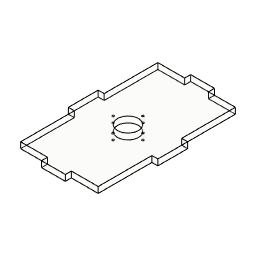
ASM_asian_hornet_trap (Autodesk Fusion 360 archive; units mm, degrees)
design "bottom_plate"
Autodesk Fusion 360 part; units mm, degrees
sketch "Esquisse1" plane through (0, 0, 0) normal (0, 0, 1) x (1, 0, 0)
  line L0 (75, -125) -> (-75, -125) construction
  line L1 (-75, -125) -> (-75, 125) construction
  line L2 (-75, 125) -> (75, 125) construction
  line L3 (75, 125) -> (75, -125) construction
  line L4 (75, -125) -> (-75, 125) construction
  line L5 (-75, -125) -> (75, 125) construction
  circle A0 centre (0, 0) radius 17.5
  circle A1 centre (0, 0) radius 25 construction
  circle A2 centre (0, 25) radius 1.6
  circle A3 centre (-25, 0) radius 1.6
  circle A4 centre (0, -25) radius 1.6
  circle A5 centre (25, 0) radius 1.6
  line L6 (0, 125) -> (0, -125)
  line L7 (-75, 0) -> (75, 0)
  line L8 (75, 125) -> (-75, 125) construction
  line L9 (-75, -125) -> (75, -125) construction
  line L10 (75, -125) -> (-75, -125) construction
  line L11 (-65, 115) -> (-65, 25)
  line L12 (-65, 25) -> (-75, 25)
  line L13 (-75, 25) -> (-75, -25)
  line L14 (-75, -25) -> (-65, -25)
  line L15 (-65, -25) -> (-65, -115)
  line L16 (65, 115) -> (65, 25)
  line L17 (65, 25) -> (75, 25)
  line L18 (75, -125) -> (75, 125) construction
  line L19 (75, -25) -> (65, -25)
  line L20 (65, -25) -> (65, -115)
  line L21 (75, 25) -> (75, -25)
  line L22 (-65, 115) -> (-20, 115)
  line L23 (-20, 115) -> (-20, 125)
  line L24 (20, 125) -> (-20, 125)
  line L25 (20, 125) -> (20, 115)
  line L26 (20, 115) -> (65, 115)
  line L27 (20, -125) -> (20, -115)
  line L28 (20, -115) -> (65, -115)
  line L29 (20, -125) -> (-20, -125)
  line L30 (-20, -115) -> (-20, -125)
  line L31 (-65, -115) -> (-20, -115)
  circle A6 centre (0, 0) radius 33.25 construction
  dimension "d1" = 150
  dimension "d2" = 250
  dimension "d3" = 35
  dimension "d5" = 3.2
  dimension "d9" = 50
  dimension "d14" = 40
  dimension "d15" = 10
  dimension "d16" = 10
  dimension "d17" = 66.5
  dimension "d18" = 50
  constraint horizontal L0
  constraint perpendicular L0 L1
  constraint parallel L0 L2
  constraint parallel L1 L3
  constraint coincident L4 A0.centre
  constraint coincident L5 A0.centre
  constraint coincident A0.centre A1.centre
  constraint coincident A1 A2.centre
  constraint coincident A1 A4.centre
  constraint coincident A1 A5.centre
  constraint equal A2 A5
  constraint equal A4 A5
  constraint equal A3 A4
  constraint midpoint L2 L6.start
  constraint midpoint L0 L6.end
  constraint midpoint L1 L7.start
  constraint midpoint L3 L7.end
  constraint coincident A2.centre L6
  constraint coincident A5.centre L7
  constraint coincident A4.centre L6
  constraint coincident A3.centre L7
  constraint coincident A1 A3.centre
  constraint symmetric L1.end L6 L2.end
  constraint symmetric L2.end L6 L1.end
  constraint symmetric L1.end L7 L0.end
  constraint symmetric L2.end L7 L0.start
  constraint symmetric L7 L2.end L0.start
  constraint symmetric L7 L1.end L0.end
  constraint perpendicular L8 L11
  constraint coincident L1 L12.end
  constraint perpendicular L1 L12
  constraint coincident L1 L13.end
  constraint perpendicular L13 L14
  constraint equal L12 L14
  constraint vertical L15
  constraint symmetric L7 L11.end L14.end
  constraint symmetric L0.end L6 L0.start
  constraint symmetric L6 L11.end L16.end
  constraint symmetric L6 L12.end L17.end
  constraint symmetric L6 L13.end L19.start
  constraint symmetric L6 L14.end L19.end
  constraint perpendicular L11 L22
  constraint coincident L8 L23.end
  constraint perpendicular L8 L23
  constraint coincident L2 L24.start
  constraint perpendicular L23 L24
  constraint perpendicular L24 L25
  constraint perpendicular L16 L26
  constraint symmetric L6 L23.end L24.start
  constraint equal L23 L25
  constraint vertical L16
  constraint symmetric L7 L11.start L15.end
  constraint symmetric L7 L22.end L30.start
  constraint symmetric L7 L23.end L29.end
  constraint symmetric L7 L24.start L27.start
  constraint symmetric L7 L25.end L27.end
  constraint symmetric L7 L16.start L20.end
  measures "d1" distance of L1.end L2.end
  measures "d2" distance of L0.end L1.end
  measures "d3" diameter of A0
  measures "d5" diameter of A2
  measures "d9" distance of L12 L14
  measures "d14" distance of L23 L25
  measures "d15" distance of L8 L22
  measures "d16" distance of L1 L11
  measures "d17" diameter of A6
  measures "d18" diameter of A1
extrude "Extrusion1" add sketch "Esquisse1" along normal blind 10 contours A0 A4 A5 L6 L7 L19 L20 L21 L27 L28 L29 | A0 A2 A5 L6 L7 L16 L17 L21 L24 L25 L26 | A0 A2 A3 L6 L7 L11 L12 L13 L22 L23 L24 | A0 A3 A4 L6 L7 L13 L14 L15 L29 L30 L31

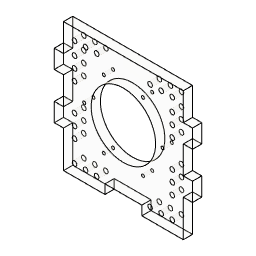
design "front_and_back_plate"
Autodesk Fusion 360 part; units mm, degrees
sketch "Esquisse1" plane through (0, 0, 0) normal (0, 1, 0) x (1, 0, 0)
  line L0 (75, 75) -> (-75, 75) construction
  line L1 (-75, 75) -> (-75, -75) construction
  line L2 (-75, -75) -> (75, -75) construction
  line L3 (75, -75) -> (75, 75) construction
  line L4 (75, 75) -> (-75, -75) construction
  line L5 (-75, 75) -> (75, -75) construction
  circle A0 centre (0, 0) radius 35
  circle A1 centre (0, 0) radius 42.5 construction
  circle A2 centre (42.5, 0) radius 1.6
  line L6 (42.5, 0) -> (21.25, 36.8061) construction
  line L7 (21.25, 36.8061) -> (-21.25, 36.8061) construction
  line L8 (-21.25, 36.8061) -> (-42.5, 0) construction
  line L9 (-42.5, 0) -> (-21.25, -36.8061) construction
  line L10 (-21.25, -36.8061) -> (21.25, -36.8061) construction
  line L11 (21.25, -36.8061) -> (42.5, 0) construction
  circle A3 centre (21.25, -36.8061) radius 1.6
  circle A4 centre (-21.25, -36.8061) radius 1.6
  circle A5 centre (-42.5, 0) radius 1.6
  circle A6 centre (-21.25, 36.8061) radius 1.6
  circle A7 centre (21.25, 36.8061) radius 1.6
  line L12 (-65, -65) -> (0, -65)
  line L13 (0, -75) -> (0, 75)
  line L14 (-75, 0) -> (75, 0)
  line L15 (65, -65) -> (0, -65)
  line L16 (-65, 65) -> (0, 65) construction
  line L17 (65, 65) -> (0, 65) construction
  line L18 (-65, 35) -> (-65, 65)
  line L19 (-65, 35) -> (-75, 35)
  line L20 (-75, -75) -> (-75, 75) construction
  line L21 (-75, 15) -> (-65, 15)
  line L22 (-65, 15) -> (-65, 0.2731)
  line L23 (75, 75) -> (75, -75) construction
  line L24 (-75, 15) -> (-75, 35)
  line L25 (-65, -65) -> (-65, -35)
  line L26 (-65, -35) -> (-75, -35)
  line L27 (-75, -15) -> (-65, -15)
  line L28 (-65, -15) -> (-65, 0.2731)
  line L29 (-65, -65) -> (-65, 75) construction
  line L30 (-75, -15) -> (-75, -35)
  line L31 (65, -15) -> (65, 0.2731)
  line L32 (65, -65) -> (65, -35)
  line L33 (75, 15) -> (75, 35)
  line L34 (65, 35) -> (75, 35)
  line L35 (75, -15) -> (75, -35)
  line L36 (75, 15) -> (65, 15)
  line L37 (65, 15) -> (65, 0.2731)
  line L38 (65, -35) -> (75, -35)
  line L39 (65, 35) -> (65, 65)
  line L40 (75, -15) -> (65, -15)
  line L41 (-65, 65) -> (-65, 75)
  line L42 (-65, 75) -> (-20, 75)
  line L43 (-20, 75) -> (-20, 65)
  line L44 (-20, 65) -> (20, 65)
  line L45 (20, 65) -> (20, 75)
  line L46 (20, 75) -> (65, 75)
  line L47 (65, 75) -> (65, 65)
  circle A8 centre (0, 0) radius 50 construction
  point P0 (75, 0)
  point P1 (-75, -25)
  point P2 (-75, 25)
  dimension "d1" = 150
  dimension "d2" = 150
  dimension "d3" = 70
  dimension "d4" = 7.5
  dimension "d5" = 3.2
  dimension "d9" = 10
  dimension "d22" = 20
  dimension "d24" = 20
  dimension "d25" = 10
  dimension "d32" = 40
  dimension "d56" = 15
  dimension "d58" = 50
  constraint horizontal L0
  constraint perpendicular L0 L1
  constraint parallel L1 L3
  constraint coincident L4 A0.centre
  constraint coincident L5 A0.centre
  constraint coincident A0.centre A1.centre
  constraint concentric A0 A1
  constraint coincident A1 A2.centre
  constraint coincident A2.centre L6.start
  constraint coincident L10.end L11.start
  constraint coincident L9.end L10.start
  constraint coincident L8.end L9.start
  constraint coincident L7.end L8.start
  constraint coincident L6.end L7.start
  constraint equal A3 A4
  constraint equal A4 A5
  constraint equal A5 A6
  constraint equal A6 A7
  constraint equal A2 A7
  constraint perpendicular L1 L12
  constraint midpoint L2 L13.start
  constraint midpoint L0 L13.end
  constraint midpoint L1 L14.start
  constraint midpoint L3 P0
  constraint symmetric L12.start L13 L15.start
  constraint symmetric L12.end L13 L15.end
  constraint symmetric L0.start L14 L2.end
  constraint symmetric L0.end L14 L1.end
  constraint symmetric L1.end L14 L0.end
  constraint symmetric L2.end L14 L0.start
  constraint symmetric L12.start L14 L16.start
  constraint symmetric L12.end L14 L16.end
  constraint symmetric L14 L15.start L17.start
  constraint symmetric L14 L12.end L16.end
  constraint coincident A2.centre L14
  constraint perpendicular L12 L25
  constraint coincident L1 L26.end
  constraint perpendicular L1 L26
  constraint coincident L1 L27.start
  constraint perpendicular L1 L27
  constraint perpendicular L14 L28
  constraint coincident L0 L29.end
  constraint perpendicular L0 L29
  constraint coincident L12.start L28
  constraint vertical L24
  constraint coincident L1 L21.start
  constraint symmetric L13 L14.start P0
  constraint symmetric L13 L16.start L17.start
  constraint symmetric L13 L18.start L34.start
  constraint symmetric L13 L19.end L33.end
  constraint symmetric L13 L21.start L33.start
  constraint symmetric L13 L21.end L36.end
  constraint symmetric L13 L22.end L31.end
  constraint symmetric L13 L25.end L32.end
  constraint symmetric L13 L26.end L35.end
  constraint symmetric L13 L27.start L35.start
  constraint symmetric L13 L27.end L31.start
  constraint vertical L22
  constraint coincident L0 L42.end
  constraint coincident L16 L43.end
  constraint perpendicular L16 L43
  constraint coincident L17 L44.end
  constraint perpendicular L43 L44
  constraint coincident L0 L45.end
  constraint perpendicular L0 L45
  constraint coincident L0 L46.end
  constraint perpendicular L17 L47
  constraint symmetric L13 L43.end L44.end
  constraint vertical L18
  constraint concentric A1 A8
  constraint symmetric L14 L21.end L27.end
  constraint midpoint L30 P1
  constraint midpoint L24 P2
  measures "d1" distance of L1.end L2.end
  measures "d2" distance of L0.end L1.end
  measures "d3" diameter of A0
  measures "d4" distance of A0 A1
  measures "d5" diameter of A3
  measures "d9" distance of L2 L12
  measures "d22" distance of L19 L21
  measures "d24" distance of L26 L27
  measures "d25" distance of L20 L29
  measures "d32" distance of L43 L45
  measures "d56" distance of A0 A8
  measures "d58" distance of P1 P2
extrude "Extrusion1" add sketch "Esquisse1" along normal blind 10 contours A0 A2 L13 L14 L15 L31 L32 L35 L38 L40 | A0 A2 L13 L14 L31 L33 L34 L36 L37 L39 L44 L45 L46 L47 | A0 A5 L13 L14 L18 L19 L21 L22 L24 L28 L41 L42 L43 L44 | A0 A5 L12 L13 L14 L25 L26 L27 L28 L30
sketch "Esquisse3" plane through (0, 0, 0) normal (0, -1, 0) x (1, 0, 0)
  line L0 (65, 65) -> (-65, 65)
  line L1 (-65, 65) -> (-65, 35)
  line L2 (-65, 35) -> (-75, 35)
  line L3 (-75, 35) -> (-75, 15)
  line L4 (-75, 15) -> (-65, 15)
  line L5 (-65, 15) -> (-65, -15)
  line L6 (-65, -15) -> (-75, -15)
  line L7 (-75, -15) -> (-75, -35)
  line L8 (-75, -35) -> (-65, -35)
  line L9 (-65, -35) -> (-65, -75)
  line L10 (-65, -75) -> (-20, -75)
  line L11 (-20, -75) -> (-20, -65)
  line L12 (-20, -65) -> (20, -65)
  line L13 (20, -65) -> (20, -75)
  line L14 (20, -75) -> (65, -75)
  line L15 (65, -75) -> (65, -35)
  line L16 (65, -35) -> (75, -35)
  line L17 (75, -35) -> (75, -15)
  line L18 (75, -15) -> (65, -15)
  line L19 (65, -15) -> (65, 15)
  line L20 (65, 15) -> (75, 15)
  line L21 (75, 15) -> (75, 35)
  line L22 (75, 35) -> (65, 35)
  line L23 (65, 35) -> (65, 65)
  circle A0 centre (-42.5, 0) radius 1.6
  circle A1 centre (21.25, 36.8061) radius 1.6
  circle A2 centre (21.25, -36.8061) radius 1.6
  circle A3 centre (-21.25, -36.8061) radius 1.6
  circle A4 centre (42.5, 0) radius 1.6
  circle A5 centre (-21.25, 36.8061) radius 1.6
  circle A6 centre (0, 0) radius 35
  line L24 (-65, -64.8) -> (65, -64.8) construction
  line L25 (-65, -62.3) -> (65, -62.3) construction
  circle A7 centre (-53, -62.3) radius 2.5
  circle A8 centre (-41, -62.3) radius 2.5
  circle A9 centre (-29, -62.3) radius 2.5
  line L26 (0, -64.8) -> (0, 65)
  circle A10 centre (41, -62.3) radius 2.5
  circle A11 centre (53, -62.3) radius 2.5
  circle A12 centre (29, -62.3) radius 2.5
  line L27 (-53, -75) -> (-53, 65) construction
  circle A13 centre (-53, -39) radius 2.5
  circle A14 centre (-53, -27) radius 2.5
  circle A15 centre (-53, -15) radius 2.5
  circle A16 centre (-53, 15) radius 2.5
  circle A17 centre (-53, 27) radius 2.5
  circle A18 centre (-53, 39) radius 2.5
  line L28 (-65, 0) -> (65, 0)
  circle A19 centre (53, -15) radius 2.5
  circle A20 centre (53, 39) radius 2.5
  circle A21 centre (53, -39) radius 2.5
  circle A22 centre (53, 15) radius 2.5
  circle A23 centre (53, 27) radius 2.5
  circle A24 centre (53, -27) radius 2.5
  line L29 (53, -75) -> (53, 65) construction
  line L30 (-53, 53) -> (53, 53) construction
  circle A25 centre (-53, 53) radius 2.5
  circle A26 centre (-41, 53) radius 2.5
  circle A27 centre (-29, 53) radius 2.5
  line L31 (-41, 53) -> (-41, -62.3) construction
  line L32 (-29, 53) -> (-29, -62.3) construction
  circle A28 centre (53, 53) radius 2.5
  circle A29 centre (29, 53) radius 2.5
  circle A30 centre (41, 53) radius 2.5
  circle A31 centre (0, 0) radius 50 construction
  point P0 (41, 53)
  point P1 (53, 53)
  point P2 (29, 53)
  dimension "d33" = 0.2
  dimension "d34" = 5
  dimension "d36" = 12
  dimension "d37" = 12
  dimension "d38" = 12
  dimension "d39" = 5
  dimension "d40" = 5
  dimension "d41" = 5
  dimension "d42" = 5
  dimension "d43" = 5
  dimension "d44" = 5
  dimension "d45" = 12
  dimension "d46" = 12
  dimension "d47" = 12
  dimension "d48" = 12
  dimension "d49" = 30
  dimension "d50" = 12
  dimension "d51" = 5
  dimension "d52" = 5
  dimension "d53" = 5
  dimension "d54" = 12
  dimension "d57" = 15
  constraint coincident L9 L24.start
  constraint coincident L15 L24.end
  constraint perpendicular L15 L24
  constraint coincident L9 L25.start
  constraint coincident L15 L25.end
  constraint perpendicular L15 L25
  constraint coincident L25 A7.centre
  constraint coincident L25 A8.centre
  constraint coincident L25 A9.centre
  constraint equal A8 A9
  constraint equal A7 A8
  constraint tangent L24 A7
  constraint midpoint L24 L26.start
  constraint midpoint L0 L26.end
  constraint symmetric A7 L26 A11
  constraint symmetric A8 L26 A10
  constraint symmetric A9 L26 A12
  constraint coincident L10 L27.start
  constraint coincident L0 L27.end
  constraint perpendicular L0 L27
  constraint coincident L27 A13.centre
  constraint coincident L27 A14.centre
  constraint coincident L27 A15.centre
  constraint coincident L27 A16.centre
  constraint coincident L27 A17.centre
  constraint coincident L27 A18.centre
  constraint midpoint L5 L28.start
  constraint midpoint L19 L28.end
  constraint symmetric A15.centre A16.centre L28
  constraint symmetric L26 L27.start L29.start
  constraint symmetric L26 L27.end L29.end
  constraint symmetric L26 A13 A21
  constraint symmetric L26 A14 A24
  constraint symmetric L26 A15 A19
  constraint symmetric L26 A16 A22
  constraint symmetric L26 A17 A23
  constraint symmetric L26 A18 A20
  constraint coincident L27 L30.start
  constraint coincident L29 P1
  constraint perpendicular L29 L30
  constraint coincident L30.start A25.centre
  constraint coincident L30 A26.centre
  constraint coincident L30 A27.centre
  constraint coincident A26.centre L31.start
  constraint coincident A8.centre L31.end
  constraint coincident A27.centre L32.start
  constraint coincident A9.centre L32.end
  constraint vertical L32
  constraint vertical L31
  constraint symmetric L26 L30.start P1
  constraint symmetric L26 A25 A28
  constraint symmetric L26 A26 A30
  constraint symmetric L26 A27 A29
  constraint symmetric L26 A26.centre P0
  constraint symmetric L26 A27.centre P2
  constraint coincident A6.centre A31.centre
  measures "d33" distance of L12 L24
  measures "d34" diameter of A7
  measures "d36" distance of A7.centre A8.centre
  measures "d37" distance of A8.centre A9.centre
  measures "d38" distance of L25.start A7.centre
  measures "d39" diameter of A13
  measures "d40" diameter of A14
  measures "d41" diameter of A15
  measures "d42" diameter of A16
  measures "d43" diameter of A17
  measures "d44" diameter of A18
  measures "d45" distance of A13.centre A14.centre
  measures "d46" distance of A14.centre A15.centre
  measures "d47" distance of A16.centre A17.centre
  measures "d48" distance of A17.centre A18.centre
  measures "d49" distance of A15.centre A16.centre
  measures "d50" distance of L1 L27
  measures "d51" diameter of A25
  measures "d52" diameter of A26
  measures "d53" diameter of A27
  measures "d54" distance of L0 L30
  measures "d57" distance of A6 A31
extrude "Extrusion3" cut sketch "Esquisse3" against normal through all contours A7 | A8 | A9 | A10 | A11 | A12 | A13 | A14 | A15 | A16 | A17 | A18 | A19 | A20 | A21 | A22 | A23 | A24 | A25 | A26 | A27 | A28 | A29 | A30

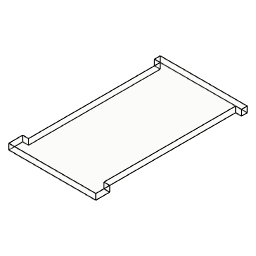
design "top_plate"
Autodesk Fusion 360 part; units mm, degrees
sketch "Esquisse1" plane through (0, 0, 0) normal (0, 0, 1) x (1, 0, 0)
  line L0 (75, -125) -> (-75, -125) construction
  line L1 (-75, -125) -> (-75, 125) construction
  line L2 (-75, 125) -> (75, 125) construction
  line L3 (75, 125) -> (75, -125) construction
  line L4 (75, -125) -> (-75, 125) construction
  line L5 (-75, -125) -> (75, 125) construction
  line L6 (-75, 125) -> (75, 125) construction
  line L7 (75, 125) -> (75, 136) construction
  line L8 (75, 136) -> (-75, 136) construction
  line L9 (-75, 136) -> (-75, 125) construction
  line L10 (-75, 136) -> (-75, 126)
  line L11 (-75, 126) -> (-65, 126)
  line L12 (-65, 126) -> (-65, -101)
  line L13 (-65, -101) -> (-75, -101)
  line L14 (-75, -101) -> (-75, -125)
  line L15 (-75, -125) -> (0, -125)
  line L16 (0, -125) -> (0, -120)
  line L17 (0, -120) -> (0, 136)
  line L18 (-75, 136) -> (0, 136)
  line L19 (75, 136) -> (0, 136)
  line L20 (75, 136) -> (75, 125) construction
  line L21 (0, -120) -> (0, 136)
  line L22 (0, -125) -> (0, -120)
  line L23 (75, -101) -> (75, -125)
  line L24 (75, -125) -> (0, -125)
  line L25 (65, -101) -> (75, -101)
  line L26 (75, -125) -> (75, 125) construction
  line L27 (75, 126) -> (65, 126)
  line L28 (75, 136) -> (75, 126)
  line L29 (65, 126) -> (65, -101)
  dimension "d1" = 150
  dimension "d2" = 250
  dimension "d3" = 11
  dimension "d4" = 10
  dimension "d5" = 10
  dimension "d6" = 24
  constraint horizontal L0
  constraint perpendicular L0 L1
  constraint parallel L0 L2
  constraint parallel L1 L3
  constraint coincident L4 origin
  constraint coincident L5 origin
  constraint horizontal L6
  constraint vertical L7
  constraint horizontal L8
  constraint vertical L9
  constraint coincident L9 L10.end
  constraint perpendicular L2 L10
  constraint perpendicular L10 L11
  constraint perpendicular L2 L12
  constraint coincident L1 L13.end
  constraint perpendicular L1 L13
  constraint midpoint L0 L15.end
  constraint perpendicular L0 L16
  constraint midpoint L8 L17.end
  constraint perpendicular L8 L17
  constraint symmetric L0.end L17 L0.start
  constraint symmetric L1.end L17 L2.end
  constraint symmetric L8.end L17 L7.end
  constraint symmetric L10.end L17 L27.start
  constraint symmetric L11.end L17 L27.end
  constraint symmetric L12.end L17 L25.start
  constraint symmetric L13.end L17 L23.start
  constraint symmetric L15.end L17 L16.start
  constraint symmetric L16.end L17 L21.start
  constraint symmetric L18.end L17 L19.end
  measures "d1" distance of L0.start L0.end
  measures "d2" distance of L0.start L2.end
  measures "d3" distance of L1.end L8.end
  measures "d4" distance of L10.end L11.end
  measures "d5" distance of L8 L11
  measures "d6" distance of L13 L15
extrude "Extrusion1" add sketch "Esquisse1" along normal blind 10

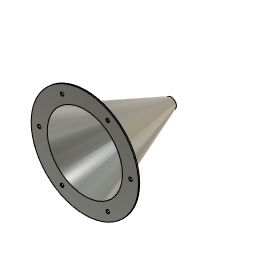
design "cone"
Autodesk Fusion 360 part; units mm, degrees
sketch "Esquisse1" plane through (0, 0, 0) normal (0, 0, 1) x (1, 0, 0)
  line L0 (0, 0) -> (0, 80)
  line L1 (0, 0) -> (50, 0) construction
  line L2 (50, 0) -> (50, 1)
  line L3 (50, 1) -> (35.685, 1)
  line L4 (35.685, 1) -> (4.9324, 80.3613)
  line L5 (4, 80) -> (35, 0)
  line L6 (35, 0) -> (50, 0)
  line L7 (4.9324, 80.3613) -> (4, 80)
  line L8 (4, 80) -> (0, 80) construction
  dimension "d1" = 1
  dimension "d2" = 35
  dimension "d3" = 15
  dimension "d4" = 4
  dimension "d5" = 80
  constraint coincident L0.start L1.start
  constraint vertical L0
  constraint perpendicular L0 L1
  constraint perpendicular L1 L2
  constraint perpendicular L2 L3
  constraint coincident L1 L5.end
  constraint parallel L4 L5
  constraint perpendicular L5 L7
  constraint horizontal L8
  constraint equal L2 L7
  measures "d1" distance of L1.end L2.end
  measures "d2" distance of L0.start L5.end
  measures "d3" distance of L1.end L5.end
  measures "d4" distance of L0.end L5.start
  measures "d5" distance of L0.start L0.end
revolve "Révolution1" add sketch "Esquisse1" angle 360 about axis through (0, 0, 0) along (0, 1, 0)
sketch "Esquisse2" plane through (0, 0, 0) normal (0, -1, 0) x (1, 0, 0)
  circle A0 centre (0, 0) radius 50
  circle A1 centre (0, 0) radius 35
  line L0 (21.25, 36.8061) -> (-21.25, 36.8061) construction
  line L1 (-21.25, 36.8061) -> (-42.5, 0) construction
  line L2 (-42.5, 0) -> (-21.25, -36.8061) construction
  line L3 (-21.25, -36.8061) -> (21.25, -36.8061) construction
  line L4 (21.25, -36.8061) -> (42.5, 0) construction
  line L5 (42.5, 0) -> (21.25, 36.8061) construction
  line L6 (-50, 0) -> (50, 0) construction
  circle A2 centre (0, 0) radius 42.5 construction
  circle A3 centre (-21.25, 36.8061) radius 1.6
  circle A4 centre (21.25, 36.8061) radius 1.6
  circle A5 centre (42.5, 0) radius 1.6
  circle A6 centre (21.25, -36.8061) radius 1.6
  circle A7 centre (-21.25, -36.8061) radius 1.6
  circle A8 centre (-42.5, 0) radius 1.6
  dimension "d7" = 7.5
  dimension "d8" = 3.2
  constraint coincident A0.centre A1.centre
  constraint coincident A0 L6.start
  constraint coincident A0 L6.end
  constraint horizontal L6
  constraint coincident L4.end L6
  constraint coincident A0.centre L6
  constraint coincident L0.end A2
  constraint coincident L0.end L1.start
  constraint coincident L0.start L5.end
  constraint coincident L4.end L5.start
  constraint coincident L3.end L4.start
  constraint coincident L2.end L3.start
  constraint coincident L1.end L2.start
  constraint equal A3 A4
  constraint equal A4 A5
  constraint equal A5 A6
  constraint equal A6 A7
  constraint equal A7 A8
  measures "d7" distance of A1 A2
  measures "d8" diameter of A3
extrude "Extrusion1" cut sketch "Esquisse2" against normal through all contours A3 | A4 | A5 | A6 | A7 | A8
equation "d2 = ( 70 / 2 ) * 1 mm"

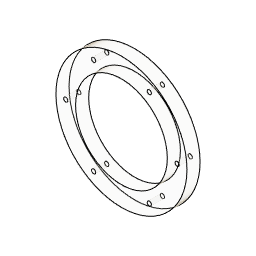
design "cone_fastener"
Autodesk Fusion 360 part; units mm, degrees
sketch "Esquisse1" plane through (0, 0, 0) normal (0, 1, 0) x (1, 0, 0)
  circle A0 centre (0, 0) radius 35
  circle A1 centre (0, 0) radius 50
  line L0 (42.5, 0) -> (21.25, 36.8061) construction
  line L1 (21.25, 36.8061) -> (-21.25, 36.8061) construction
  line L2 (-21.25, 36.8061) -> (-42.5, 0) construction
  line L3 (-42.5, 0) -> (-21.25, -36.8061) construction
  line L4 (-21.25, -36.8061) -> (21.25, -36.8061) construction
  line L5 (21.25, -36.8061) -> (42.5, 0) construction
  circle A2 centre (0, 0) radius 42.5 construction
  line L6 (50, 0) -> (-50, 0)
  line L7 (0, -50) -> (0, 50)
  circle A3 centre (21.25, -36.8061) radius 1.6
  circle A4 centre (-21.25, -36.8061) radius 1.6
  circle A5 centre (-42.5, 0) radius 1.6
  circle A6 centre (-21.25, 36.8061) radius 1.6
  circle A7 centre (21.25, 36.8061) radius 1.6
  circle A8 centre (42.5, 0) radius 1.6
  dimension "d1" = 70
  dimension "d2" = 15
  dimension "d5" = 7.5
  dimension "d6" = 3.2
  constraint coincident A0.centre A1.centre
  constraint coincident L4.end A2
  constraint coincident A1 L6.start
  constraint coincident A1 L6.end
  constraint horizontal L6
  constraint coincident A1 L7.start
  constraint coincident A1 L7.end
  constraint perpendicular L6 L7
  constraint coincident L0.start L6
  constraint coincident L4.end L5.start
  constraint coincident L3.end L4.start
  constraint coincident A0.centre L6
  constraint coincident L2.end L3.start
  constraint coincident L1.end L2.start
  constraint coincident L0.end L1.start
  constraint coincident L0.start L5.end
  constraint equal A3 A4
  constraint equal A3 A8
  constraint equal A7 A8
  constraint equal A4 A5
  constraint equal A6 A7
  measures "d1" diameter of A0
  measures "d2" distance of A0 A1
  measures "d5" distance of A0 A2
  measures "d6" diameter of A4
extrude "Extrusion1" add sketch "Esquisse1" along normal blind 10 contours A0 A1 L6 L7 A8 | A0 A1 L6 L7 A8 | A0 A1 L6 L7 A5 | A0 A1 L6 L7 A5

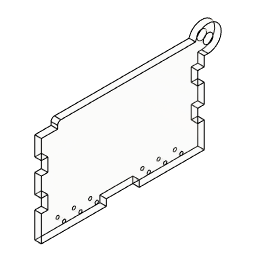
design "right_and_left_plate"
Autodesk Fusion 360 part; units mm, degrees
sketch "Esquisse1" plane through (0, 0, 0) normal (1, 0, 0) x (0, 1, 0)
  line L0 (0, 0) -> (-250, 0) construction
  line L1 (-250, 0) -> (-250, 150) construction
  line L2 (-220, 150) -> (0, 150) construction
  line L3 (0, 150) -> (0, 0) construction
  line L4 (0, 0) -> (0, 39.75)
  line L5 (-10, 39.75) -> (0, 39.75)
  line L6 (-10, 39.75) -> (-10, 60.25)
  line L7 (-10, 60.25) -> (0, 60.25)
  line L8 (0, 60.25) -> (0, 89.75)
  line L9 (-10, 89.75) -> (-10, 110.25)
  line L10 (-10, 110.25) -> (0, 110.25)
  line L11 (-10, 89.75) -> (0, 89.75)
  line L12 (0, 110.25) -> (0, 125)
  line L13 (-13.3649, 150) -> (-250, 150) construction
  line L14 (11, 150) -> (1, 150) construction
  line L15 (1, 150) -> (1, 140) construction
  line L16 (1, 140) -> (11, 140) construction
  line L17 (11, 140) -> (11, 150) construction
  line L18 (11, 150) -> (1, 140) construction
  line L19 (1, 150) -> (11, 140) construction
  arc A0 (6, 125) -> (-13.3649, 150) centre (6, 145) ccw
  line L20 (-13.3649, 150) -> (-220, 150)
  line L21 (-250, 140) -> (-250, 110.5)
  line L22 (-250, 110.5) -> (-240, 110.5)
  line L23 (-240, 110.5) -> (-240, 90)
  line L24 (-240, 90) -> (-250, 90)
  line L25 (-250, 90) -> (-250, 60.5)
  line L26 (-250, 60.5) -> (-240, 60.5)
  line L27 (-240, 60.5) -> (-240, 40)
  line L28 (-240, 40) -> (-250, 40)
  line L29 (-250, 40) -> (-250, 0)
  line L30 (-250, 0) -> (-150.25, 0)
  line L31 (-150.25, 0) -> (-150.25, 10)
  line L32 (-150.25, 10) -> (-99.75, 10)
  line L33 (-99.75, 10) -> (-99.75, 0)
  line L34 (-99.75, 0) -> (0, 0)
  line L35 (-125, 150) -> (-125, 10) construction
  line L36 (-250, 75) -> (0, 75) construction
  circle A1 centre (6, 145) radius 7.5
  circle A2 centre (6, 145) radius 7.0711 construction
  line L37 (-125, 150) -> (-125, 0) construction
  line L38 (-225, 145) -> (-225, 140)
  line L39 (-225, 140) -> (-250, 140)
  line L40 (0, 140) -> (-250, 140) construction
  line L41 (0, 125) -> (6, 125)
  arc A3 (6, 125) -> (0, 125.9212) centre (6, 145) ccw construction
  arc A4 (0, 125.9212) -> (6, 125) centre (6, 145) ccw construction
  arc A5 (-220, 150) -> (-225, 145) centre (-220, 145) ccw
  point P0 (6, 145)
  point P1 (-10, 100)
  point P2 (-10, 50)
  dimension "d1" = 250
  dimension "d2" = 150
  dimension "d4" = 20.5
  dimension "d7" = 10
  dimension "d8" = 40
  dimension "d11" = 10
  dimension "d12" = 10
  dimension "d13" = 40
  dimension "d29" = 50.5
  dimension "d30" = 10
  dimension "d36" = 140
  dimension "d37" = 10
  dimension "d38" = 1
  dimension "d40" = 5
  dimension "d41" = 50
  dimension "d42" = 15
  dimension "d43" = 25
  constraint horizontal L0
  constraint vertical L1
  constraint horizontal L2
  constraint vertical L3
  constraint coincident L0.start L3.end
  constraint coincident L3 L4.end
  constraint perpendicular L3 L5
  constraint perpendicular L5 L6
  constraint coincident L3 L7.end
  constraint perpendicular L3 L7
  constraint coincident L3 L8.end
  constraint perpendicular L7 L9
  constraint coincident L3 L10.end
  constraint perpendicular L3 L10
  constraint perpendicular L3 L11
  constraint coincident L3 A3.end
  constraint equal L7 L11
  constraint coincident L13.start A3
  constraint coincident L2 L13.start
  constraint horizontal L14
  constraint perpendicular L14 L15
  constraint parallel L14 L16
  constraint parallel L15 L17
  constraint coincident L18 P0
  constraint coincident L19 P0
  constraint coincident P0 A0.centre
  constraint equal A0 A3
  constraint coincident L1 L21.end
  constraint perpendicular L21 L22
  constraint perpendicular L22 L23
  constraint coincident L1 L24.end
  constraint perpendicular L1 L24
  constraint coincident L1 L25.end
  constraint perpendicular L1 L26
  constraint perpendicular L26 L27
  constraint coincident L1 L28.end
  constraint perpendicular L1 L28
  constraint perpendicular L0 L29
  constraint coincident L0 L30.end
  constraint perpendicular L30 L31
  constraint perpendicular L31 L32
  constraint coincident L0 L33.end
  constraint perpendicular L0 L33
  constraint equal L10 L22
  constraint equal L9 L23
  constraint equal L8 L25
  constraint equal L6 L27
  constraint equal L24 L26
  constraint midpoint L32 L35.end
  constraint vertical L35
  constraint midpoint L1 L36.start
  constraint midpoint L8 L36.end
  constraint concentric A0 A1
  constraint coincident L14.start A2
  constraint midpoint L0 L37.end
  constraint coincident L35 L37.start
  constraint coincident L13 L35.start
  constraint perpendicular L20 L38
  constraint perpendicular L38 L39
  constraint coincident L3 L40.start
  constraint coincident L1 L21.start
  constraint horizontal L40
  constraint coincident L3 L12.end
  constraint tangent A0 L41
  constraint horizontal L41
  constraint concentric A0 A4
  constraint coincident L2 L35.start
  constraint coincident L1.end L2
  constraint tangent L38 A5
  constraint tangent L2 A5
  constraint vertical L37
  constraint equal L6 L9
  constraint symmetric L7.end L8.end L36
  constraint midpoint L9 P1
  constraint midpoint L6 P2
  constraint coincident L39 L21.start
  constraint vertical L21
  measures "d1" distance of L0.start L0.end
  measures "d2" distance of L0.start L2.end
  measures "d4" distance of L5 L7
  measures "d7" distance of L3 L6
  measures "d8" diameter of A3
  measures "d11" distance of L15.end L16.end
  measures "d12" distance of L14.end L15.end
  measures "d13" distance of L0 L27.end
  measures "d29" distance of L31.end L32.end
  measures "d30" distance of L0 L32
  measures "d36" distance of L0 L40
  measures "d37" distance of L2 L16
  measures "d38" distance of L3 L15
  measures "d40" radius of A5
  measures "d41" distance of P1 P2
  measures "d42" diameter of A1
  measures "d43" distance of L38.end L21.start
extrude "Extrusion1" add sketch "Esquisse1" along normal blind 10
sketch "Esquisse2" plane through (10, 0, 0) normal (1, 0, 0) x (0, 1, 0)
  circle A0 centre (6, 145) radius 7.5
  line L0 (-250, 140) -> (-250, 110.5)
  line L1 (-250, 110.5) -> (-240, 110.5)
  line L2 (-240, 110.5) -> (-240, 90)
  line L3 (-240, 90) -> (-250, 90)
  line L4 (-250, 90) -> (-250, 60.5)
  line L5 (-250, 60.5) -> (-240, 60.5)
  line L6 (-240, 60.5) -> (-240, 40)
  line L7 (-240, 40) -> (-250, 40)
  line L8 (-250, 40) -> (-250, 0)
  line L9 (-250, 0) -> (-150.25, 0)
  line L10 (-150.25, 0) -> (-150.25, 10)
  line L11 (-150.25, 10) -> (-99.75, 10)
  line L12 (-99.75, 10) -> (-99.75, 0)
  line L13 (-99.75, 0) -> (0, 0)
  line L14 (0, 0) -> (0, 39.75)
  line L15 (0, 39.75) -> (-10, 39.75)
  line L16 (-10, 39.75) -> (-10, 60.25)
  line L17 (-10, 60.25) -> (0, 60.25)
  line L18 (0, 60.25) -> (0, 89.75)
  line L19 (0, 89.75) -> (-10, 89.75)
  line L20 (-10, 89.75) -> (-10, 110.25)
  line L21 (-10, 110.25) -> (0, 110.25)
  line L22 (0, 110.25) -> (0, 125)
  arc A1 (6, 125) -> (-13.3649, 150) centre (6, 145) ccw
  line L23 (-13.3649, 150) -> (-220, 150)
  line L24 (-250, 12.7) -> (0, 12.7) construction
  circle A2 centre (-215, 12.7) radius 2.5
  circle A3 centre (-190, 12.7) radius 2.5
  circle A4 centre (-165, 12.7) radius 2.5
  line L25 (-250, 10.2) -> (0, 10.2) construction
  line L26 (-125, 140) -> (-125, 10)
  circle A5 centre (-35, 12.7) radius 2.5
  circle A6 centre (-85, 12.7) radius 2.5
  circle A7 centre (-60, 12.7) radius 2.5
  line L27 (-225, 145) -> (-225, 140)
  line L28 (-225, 140) -> (-250, 140)
  line L29 (0, 125) -> (6, 125)
  arc A8 (-220, 150) -> (-225, 145) centre (-220, 145) ccw
  point P0 (0, 12.7)
  point P1 (0, 10.2)
  dimension "d22" = 5
  dimension "d24" = 0.2
  dimension "d25" = 25
  dimension "d26" = 25
  dimension "d27" = 35
  constraint coincident L8 L24.start
  constraint coincident L14 P0
  constraint perpendicular L14 L24
  constraint coincident L24 A2.centre
  constraint coincident L24 A3.centre
  constraint coincident L24 A4.centre
  constraint equal A3 A4
  constraint equal A2 A3
  constraint coincident L8 L25.start
  constraint coincident L14 P1
  constraint perpendicular L14 L25
  constraint tangent A2 L25
  constraint midpoint L11 L26.end
  constraint symmetric L24.start L26 P0
  constraint symmetric A2 L26 A5
  constraint symmetric A3 L26 A7
  constraint symmetric A4 L26 A6
  constraint symmetric L25.start L26 P1
  measures "d22" diameter of A2
  measures "d24" distance of L11 L25
  measures "d25" distance of A2.centre A3.centre
  measures "d26" distance of A3.centre A4.centre
  measures "d27" distance of L8 A2.centre
extrude "Extrusion2" cut sketch "Esquisse2" against normal through all contours A2 | A3 | A4 | A5 | A6 | A7
